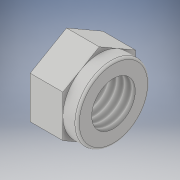
# Autodesk Inventor part: Nut 4mm self locking
Saved by Autodesk Inventor 2018 (Build 220112000, 112)
## iProperties
Created: 2018-06-26
Part Number: Nut 4mm self locking
Material: Generic
Document SubType Name: Modeling
Designer: Ajith Thomas
Density: 1 g/cm^3
Appearance: Default
Author: Ajith Thomas
Autodesk Inventor part; units mm, degrees
ref_plane "YZ Plane" through (0, 0, 0) normal (1, 0, 0) x (0, 1, 0)
ref_plane "XZ Plane" through (0, 0, 0) normal (0, 1, 0) x (-1, 0, 0)
ref_plane "XY Plane" through (0, 0, 0) normal (0, 0, 1) x (1, 0, 0)
sketch "Sketch1" plane through (0, 0, 0) normal (1, 0, 0) x (0, 1, 0)
  circle A0 centre (0, 0) radius 3.85 construction
  line L0 (-3.85, 0) -> (-1.925, 3.3342)
  line L1 (-1.925, 3.3342) -> (1.925, 3.3342)
  line L2 (1.925, 3.3342) -> (3.85, 0)
  line L3 (3.85, 0) -> (1.925, -3.3342)
  line L4 (1.925, -3.3342) -> (-1.925, -3.3342)
  line L5 (-1.925, -3.3342) -> (-3.85, 0)
  circle A1 centre (0, 0) radius 2
  dimension "d0" = 7.7
  dimension "d1" = 4
  constraints: 12 end point, 3 coincident, 1 centre point, 1 horizontal alignment, 15 other
  measures "d1" diameter of A1
extrude "Extrusion1" add sketch "Sketch1" along normal mid plane 3
sketch "Sketch2" plane through (1.5, 0, 0) normal (1, 0, 0) x (0, 0, -1)
  circle A0 centre (0, 0) radius 3.3342
  circle A1 centre (0, 0) radius 2
  constraints: 2 centre point, 2 coincident
extrude "Extrusion2" add sketch "Sketch2" along normal blind 1.3
fillet "Fillet1" radius 0.2 1 edges at (2.8, 0, 3.3342)
thread "Thread1" size "M4x0.7" class "6H" standard "ANSI Metric M Profile" full length
body "Solid1"
